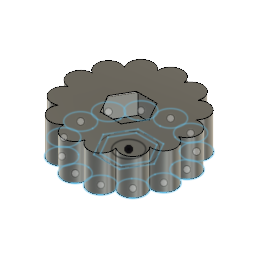
WingedNutThroughScrew v3 (Autodesk Fusion 360 design; units mm, degrees)
Autodesk Fusion 360 part; units mm, degrees
sketch "Sketch1" plane through (0, 0, 0) normal (0, 0, 1) x (1, 0, 0)
  circle A0 centre (0, 0) radius 1.5
  circle A1 centre (0, 0) radius 2.75 construction
  line L0 (1.5877, -2.75) -> (3.1754, 0)
  line L1 (3.1754, 0) -> (1.5877, 2.75)
  line L2 (1.5877, 2.75) -> (-1.5877, 2.75)
  line L3 (-1.5877, 2.75) -> (-3.1754, 0)
  line L4 (-3.1754, 0) -> (-1.5877, -2.75)
  line L5 (-1.5877, -2.75) -> (1.5877, -2.75)
  circle A2 centre (-6, 0) radius 1.5
  circle A3 centre (-5.3127, -2.7883) radius 1.5
  circle A4 centre (-3.4084, -4.9379) radius 1.5
  circle A5 centre (-0.7232, -5.9563) radius 1.5
  circle A6 centre (2.1276, -5.6101) radius 1.5
  circle A7 centre (4.4911, -3.9787) radius 1.5
  circle A8 centre (5.8257, -1.4359) radius 1.5
  circle A9 centre (5.8257, 1.4359) radius 1.5
  circle A10 centre (4.4911, 3.9787) radius 1.5
  circle A11 centre (2.1276, 5.6101) radius 1.5
  circle A12 centre (-0.7232, 5.9563) radius 1.5
  circle A13 centre (-3.4084, 4.9379) radius 1.5
  circle A14 centre (-5.3127, 2.7883) radius 1.5
  line L6 (-1.2902, 2.2348) -> (-2.5805, 0)
  line L7 (-2.5805, 0) -> (-1.2902, -2.2348)
  line L8 (-1.2902, -2.2348) -> (1.2902, -2.2348)
  line L9 (1.2902, -2.2348) -> (2.5805, 0)
  line L10 (2.5805, 0) -> (1.2902, 2.2348)
  line L11 (1.2902, 2.2348) -> (-1.2902, 2.2348)
  dimension "d6" = 3
  dimension "d7" = 5.5
  dimension "d8" = 3
  dimension "d10" = 6
  dimension "d12" = 360
  constraint coincident A0.centre A1.centre
  constraint concentric A0 A1
  measures "d6" diameter of A0
  measures "d7" diameter of A1
  measures "d8" diameter of A2
  measures "d10" distance of A0.centre A2.centre
extrude "Extrude1" add sketch "Sketch1" along normal blind 4.5 contours A0 | L0 L1 L2 L3 L4 L5 | A2 A3 A14 | A2 A3 A4 A5 A6 A7 A8 A9 A10 A11 A12 A13 A14 | A2 A14 | A2 A13 A14 | A2 A3 A4 | A2 A3 | A13 A14 | A12 A13 A14 | A3 A4 | A3 A4 A5 | A12 A13 | A11 A12 A13 | A4 A5 | A4 A5 A6 | A11 A12 | A10 A11 A12 | A5 A6 | A5 A6 A7 | A10 A11 | A9 A10 A11 | A6 A7 A8 | A6 A7 | A8 A9 A10 | A9 A10 | A7 A8 A9 | A7 A8 | A8 A9 | L6 L7 L8 L9 L10 L11
extrude "Extrude2" cut sketch "Sketch1" along normal blind 4.5 contours A0
extrude "Extrude3" cut sketch "Sketch1" along normal blind 3 from surface at 1.5 contours L0 L1 L2 L3 L4 L5 | L6 L7 L8 L9 L10 L11
extrude "Extrude4" add sketch "Sketch1" along normal blind 0.5 from surface at 4 contours L0 L1 L2 L3 L4 L5
fillet "Fillet2" radius 1 6 edges at (0, 2.2348, 4) (-1.9354, 1.1174, 4) (1.9354, 1.1174, 4) (-1.9354, -1.1174, 4) (0, -2.2348, 4) (1.9354, -1.1174, 4)
equation "screwDiam = 3 mm"
equation "FlatSideNutDistance = 5.5 mm"
equation "solidBaseHeight = 1.5 mm"
equation "totalHeight = 4.5 mm"
equation "wingDiameter = 12 mm"
equation "d6 = screwDiam"
equation "d7 = FlatSideNutDistance"
equation "d10 = wingDiameter / 2"
equation "d11 = bumpCicles"
equation "d12 = 360.00 °"
equation "bumpCicles = 13"
equation "d14 = totalHeight"
equation "d16 = totalHeight"
equation "d18 = solidBaseHeight"
equation "d19 = totalHeight - solidBaseHeight"
equation "d22 = totalHeight - 0.5 mm"
named bodies: "wing"
